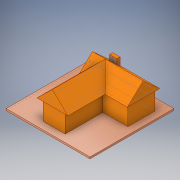
# Autodesk Inventor part: house_1
Saved by Autodesk Inventor 2019 (Build 230136000, 136)
## iProperties
Created: 2020-04-29
Part Number: house_1
Material: Wood (Oak)
Document SubType Name: Modeling
Designer: infinity
Density: 0.76 g/cm^3
Appearance: White Oak - Natural Medium Gloss
Author: infinity
Autodesk Inventor part; units mm, degrees
ref_plane "YZ Plane" through (0, 0, 0) normal (1, 0, 0) x (0, 1, 0)
ref_plane "XZ Plane" through (0, 0, 0) normal (0, 1, 0) x (-1, 0, 0)
ref_plane "XY Plane" through (0, 0, 0) normal (0, 0, 1) x (1, 0, 0)
sketch "Sketch1" plane through (0, 0, 0) normal (0, 1, 0) x (-1, 0, 0)
  line L0 (0, 0) -> (1219.2, 0)
  line L1 (1219.2, 0) -> (1219.2, -1219.2)
  line L2 (1219.2, -1219.2) -> (0, -1219.2)
  line L3 (0, -1219.2) -> (0, 0)
  dimension "d0" = 1219.2
  dimension "d1" = 1219.2
  constraints: 8 end point, 2 parallel, 1 horizontal, 1 perpendicular
  measures "d0" distance of L0.end L1.end
  measures "d1" distance of L1.end L2.end
extrude "Extrusion1" add sketch "Sketch1" along normal blind 25.4
sketch "Sketch2" plane through (0, 25.4, 0) normal (0, 1, 0) x (1, 0, 0)
  line L0 (-790.7708, 108.1811) -> (-790.7708, 1049.4054)
  line L1 (-790.7708, 1049.4054) -> (-104.9708, 1049.4054)
  line L2 (-104.9708, 1049.4054) -> (-104.9708, 656.4029)
  line L3 (-104.9708, 656.4029) -> (-468.5932, 656.4029)
  line L4 (-468.5932, 656.4029) -> (-468.5932, 108.1811)
  line L5 (-468.5932, 108.1811) -> (-790.7708, 108.1811)
  point P0 (0, 0)
  dimension "d10" = 685.8
  constraints: 12 end point, 5 perpendicular, 1 vertical
  measures "d10" distance of L0.end L1.end
extrude "Extrusion2" add sketch "Sketch2" along normal blind 304.8
sketch "Sketch3" plane through (-104.9708, 25.4, -656.4029) normal (1, 0, 0) x (0, 0, -1)
  line L0 (-33.1569, 274.7838) -> (196.5012, 492.1801)
  line L1 (196.5012, 492.1801) -> (437.777, 274.7838)
  line L2 (437.777, 274.7838) -> (-33.1569, 274.7838)
  line L3 (0, 304.8) -> (393.0024, 304.8) projected
  point P0 (-656.4029, -25.4)
  constraints: 6 end point, 1 parallel
extrude "Extrusion3" add sketch "Sketch3" along normal blind 25.4
extrude "Extrusion4" add sketch "Sketch3" against normal blind 711.2
sketch "Sketch4" plane through (-790.7708, 25.4, -108.1811) normal (0, 0, 1) x (1, 0, 0)
  line L0 (-63.4257, 274.7838) -> (161.0888, 492.1801)
  line L1 (161.0888, 492.1801) -> (386.3126, 274.7838)
  line L2 (322.1776, 274.7838) -> (711.2, 274.7838) projected
  line L3 (-63.4257, 274.7838) -> (386.3126, 274.7838)
  line L4 (0, 304.8) -> (322.1776, 304.8) projected
  line L5 (711.2, 492.1801) -> (-25.4, 492.1801) projected
  point P0 (790.7708, -25.4)
  constraints: 6 end point, 2 point on line, 1 parallel
extrude "Extrusion5" add sketch "Sketch4" against normal blind 744.22
extrude "Extrusion6" add sketch "Sketch4" along normal blind 25.4
sketch "Sketch5" plane through (0, 0, 0) normal (0, -1, 0) x (1, 0, 0)
  line L0 (-560.0074, -996.6268) -> (-666.9511, -996.6268)
  line L1 (-666.9511, -996.6268) -> (-666.9511, -948.1994)
  line L2 (-666.9511, -948.1994) -> (-560.0074, -948.1994)
  line L3 (-560.0074, -948.1994) -> (-560.0074, -996.6268)
  point P0 (0, 0)
  constraints: 8 end point, 2 parallel, 1 horizontal, 1 perpendicular
extrude "Extrusion7" add sketch "Sketch5" against normal blind 508
equation "\"d1\" = d0"
body "Solid1"
